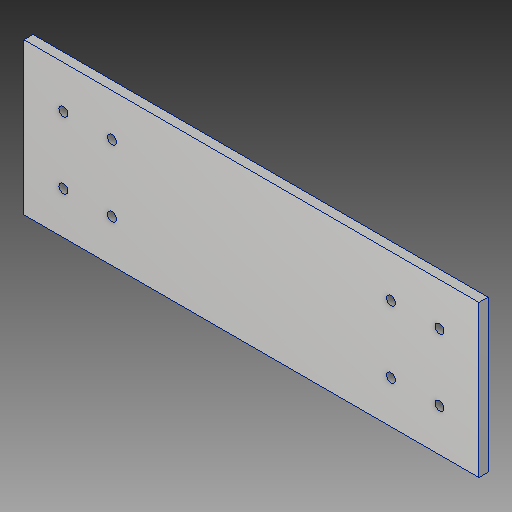
# Autodesk Inventor part: Podstawa
Saved by Autodesk Inventor 2018 (Build 220112000, 112)
## iProperties
Created: 2018-08-11
Part Number: Podstawa
Material: Ogólny
Document SubType Name: Modeling
Designer: Wojciech
Density: 1 g/cm^3
Appearance: Aluminium — płaski
Mass: 22.3304 g
Surface Area: 163.131 cm^2
Volume: 22.3304 cm^3
Author: Wojciech
Autodesk Inventor part; units mm, degrees
ref_plane "YZ Plane" through (0, 0, 0) normal (1, 0, 0) x (0, 1, 0)
ref_plane "XZ Plane" through (0, 0, 0) normal (0, 1, 0) x (-1, 0, 0)
ref_plane "XY Plane" through (0, 0, 0) normal (0, 0, 1) x (1, 0, 0)
sketch "Szkic1" plane through (0, 0, 0) normal (0, 0, 1) x (1, 0, 0)
  line L0 (-75, -25) -> (75, -25)
  line L1 (75, -25) -> (75, 25)
  line L2 (75, 25) -> (-75, 25)
  line L3 (-75, 25) -> (-75, -25)
  line L4 (-75, -25) -> (75, 25) construction
  line L5 (75, -25) -> (-75, 25) construction
  point P0 (0, 0)
  dimension "d0" = 150
  dimension "d1" = 50
  constraints: 12 end point, 2 midpoint, 2 parallel, 1 horizontal, 1 perpendicular
  measures "d0" distance of L2.end L1.end
  measures "d1" distance of L1.end L0.end
extrude "Wyciągnięcie proste1" add sketch "Szkic1" along normal blind 3
sketch "Szkic2" plane through (0, 0, 3) normal (0, 0, 1) x (1, 0, 0)
  line L0 (75, -25) -> (75, 25) projected
  line L1 (75, 25) -> (-75, 25) projected
  line L2 (-75, 25) -> (-75, -25) projected
  line L3 (-75, 0) -> (75, 0) construction
  line L4 (75, 25) -> (-75, 25) projected
  line L5 (0, 25) -> (0, -25) construction
  point P0 (0, 0)
  point P1 (62, 11)
  point P2 (46, 11)
  point P3 (62, -11)
  point P4 (46, -11)
  point P5 (-62, 11)
  point P6 (-46, 11)
  point P7 (-46, -11)
  point P8 (-62, -11)
  dimension "d4" = 13
  dimension "d5" = 16
  dimension "d6" = 14
  dimension "d7" = 14
  constraints: 6 symmetric about line, 4 end point, 3 midpoint, 1 vertical
  measures "d4" distance from line of L0 point (62, 11)
  measures "d5" distance of point (62, 11) point (46, 11)
  measures "d6" distance from line of L1 point (46, 11)
  measures "d7" distance from line of L1 point (62, 11)
hole "Otwór1" at (62, 11, 3) at (46, 11, 3) at (46, -11, 3) at (62, -11, 3) at (-46, 11, 3) at (-62, 11, 3) at (-46, -11, 3) at (-62, -11, 3) direction (0, 0, -1) diameter 3 depth 8 tip angle 118
